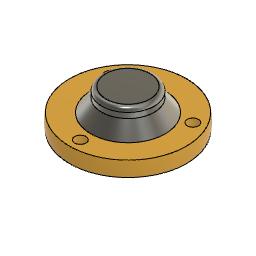
roulette_a_bille (Autodesk Fusion 360 design; units mm, degrees)
Autodesk Fusion 360 part; units mm, degrees
sketch "Esquisse1" plane through (0, 0, 0) normal (0, 0, 1) x (1, 0, 0)
  circle A0 centre (0, 0) radius 15.5
  circle A1 centre (-0.0369, -12.6) radius 1.5
  circle A2 centre (10.9304, 6.268) radius 1.5
  circle A3 centre (-10.8935, 6.332) radius 1.5
  dimension "d1" = 31
  dimension "d2" = 3
  dimension "d3" = 12.6
  dimension "d5" = 360
  constraint coincident A0.centre origin
  measures "d1" diameter of A0
  measures "d2" diameter of A1
  measures "d3" vertical distance of A0.centre A1.centre
extrude "Extrusion1" add sketch "Esquisse1" along normal mid plane 4 makes body 1
sketch "Esquisse2" plane through (0, 0, 0) normal (1, 0, 0) x (0, 1, 0)
  ellipse E0 centre (15.5, 0) end of major axis (15.5, 2) minor radius 0.25
  line L0 (15.5, -1.9999) -> (15.5, 2)
  line L1 (15.75, 0) -> (15.25, 0)
  dimension "d8" = 0.5
  dimension "d9" = 15.5
  constraint vertical L0
  constraint coincident E0 L0.start
  constraint coincident E0 L0.end
  constraint coincident E0 L1.start
  constraint coincident E0 L1.end
  measures "d9" distance of origin E0.centre
revolve "Révolution1" add sketch "Esquisse2" angle 360 about axis through (0, 0, 1.75) along (0, 0, 1) bodies 1
sketch "Esquisse3" plane through (0, 0, 2) normal (0, 0, 1) x (-1, 0, 0)
  circle A0 centre (10.8935, -6.332) radius 1.5
  circle A1 centre (0.0369, 12.6) radius 1.5
  circle A2 centre (-10.9304, -6.268) radius 1.5
  circle A3 centre (0, 0) radius 15.5
  circle A4 centre (0, 0) radius 9.85
  dimension "d11" = 19.7
  constraint coincident A3.centre A4.centre
  measures "d11" diameter of A4
extrude "Extrusion2" add sketch "Esquisse3" along normal blind 3.5 draft -39.644 contours A4 bodies 1
extrude "Extrusion3" add 1 faces at (-1.4703, -2.1565, 5.5) along direction (0, 0, 1) blind 2.5 on bodies 1 bodies 1
fillet "Congé1" radius 1.1 1 edges at (6.4797, 2.5132, 8) on bodies 1
sketch "Esquisse4" plane through (0, 0, -2) normal (0, 0, -1) x (1, 0, 0)
  circle A0 centre (-10.8935, -6.332) radius 1.5
  circle A1 centre (-0.0369, 12.6) radius 1.5
  circle A2 centre (10.9304, -6.268) radius 1.5
  circle A3 centre (0, 0) radius 15.5
sphere "SpherePrimitive3" add diameter 20 placed x (0, 1, 0) y (0, 0, 1) z (1, 0, 0) at (0, 0, 0) separate body makes body 2
split "Scinder1" by plane through (0, 0, -2) normal (0, 0, -1) bodies 2 makes body 3 at (1.8684, 9.1763, -3.5078)
delete_body "RemoveBody1" bodies 2
sphere "SpherePrimitive4" add diameter 14.3 placed x (0, 1, 0) y (0, 0, 1) z (1, 0, 0) at (0, 0, -4) separate body makes body 4
other "SpherePrimitive1"
other "SpherePrimitive2"
